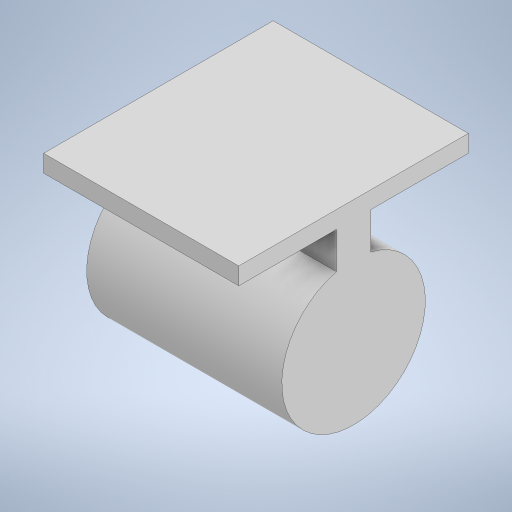
# Autodesk Inventor part: boba
Saved by Autodesk Inventor 2024 (Build 280153020, 153B)
## iProperties
Created: 2023-06-14
Part Number: boba
Material: Genérico
Document SubType Name: Modeling
Designer: victo
Density: 1 g/cm^3
Appearance: Padrão
Author: victo
Autodesk Inventor part; units mm, degrees
ref_plane "YZ Plane" through (0, 0, 0) normal (1, 0, 0) x (0, 1, 0)
ref_plane "XZ Plane" through (0, 0, 0) normal (0, 1, 0) x (-1, 0, 0)
ref_plane "XY Plane" through (0, 0, 0) normal (0, 0, 1) x (1, 0, 0)
sketch "Esboço1" plane through (0, 0, 0) normal (1, 0, 0) x (0, 1, 0)
  arc A0 (24.6347, 5.5491) -> (24.6347, -0.4509) centre (12.5, 2.5491) ccw
  line L0 (34, 2.5491) -> (34, 17.5491)
  line L1 (34, 2.5491) -> (34, -12.4509)
  line L2 (31, 5.5491) -> (24.6347, 5.5491)
  line L3 (31, -0.4509) -> (24.6347, -0.4509)
  line L4 (31, 17.5491) -> (31, 5.5491)
  line L5 (31, -0.4509) -> (31, -12.4509)
  line L6 (34, 17.5491) -> (34, 22.5491)
  line L7 (31, 17.5491) -> (31, 22.5491)
  line L8 (31, 22.5491) -> (34, 22.5491)
  line L9 (34, -12.4509) -> (34, -17.4509)
  line L10 (34, -17.4509) -> (31, -17.4509)
  line L11 (31, -17.4509) -> (31, -12.4509)
  point P0 (0, 0)
  dimension "d2" = 25
  dimension "d4" = 15
  dimension "d7" = 3
  dimension "d10" = 5
  dimension "d11" = 5
  constraints: 24 end point, 5 vertical, 4 perpendicular, 2 point on circle, 2 point on line, 1 centre point
  measures "d2" diameter of A0
  measures "d4" distance of L0.start L1.end
  measures "d7" distance of L0.end L4.start
  measures "d10" distance of L0.end L6.end
  measures "d11" distance of L1.end L9.end
extrude "Extrusão2" add sketch "Esboço1" along normal blind 34
